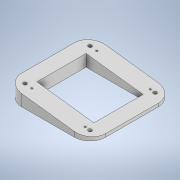
# Autodesk Inventor part: 頸部桌面轉接件
Saved by Autodesk Inventor 2021 (Build 250183000, 183)
## iProperties
Created: 2023-02-10
Part Number: 頸部桌面轉接件
Material: 一般
Document SubType Name: Modeling
Designer: brian
Density: 1 g/cm^3
Appearance: 預設
Author: brian
Autodesk Inventor part; units mm, degrees
ref_plane "YZ Plane" through (0, 0, 0) normal (1, 0, 0) x (0, 1, 0)
ref_plane "XZ Plane" through (0, 0, 0) normal (0, 1, 0) x (-1, 0, 0)
sketch "草圖1" plane through (0, 0, 0) normal (0, 1, 0) x (-1, 0, 0)
  line L0 (132.5, 132.5) -> (-132.5, 132.5)
  line L1 (-132.5, 132.5) -> (-132.5, -132.5)
  line L2 (-132.5, -132.5) -> (132.5, -132.5)
  line L3 (132.5, -132.5) -> (132.5, 132.5)
  line L4 (132.5, 132.5) -> (-132.5, -132.5) construction
  line L5 (-132.5, 132.5) -> (132.5, -132.5) construction
  point P0 (0, 0)
  dimension "d0" = 265
  dimension "d1" = 265
  constraints: 12 end point, 2 midpoint, 2 parallel, 1 horizontal, 1 perpendicular
  measures "d0" distance of L1.end L2.end
  measures "d1" distance of L0.end L1.end
extrude "擠出1" add sketch "草圖1" along normal blind 10
sketch "草圖3" plane through (0, 10, 0) normal (0, 1, 0) x (1, 0, 0)
  line L0 (132.5, -132.5) -> (132.5, 132.5) projected
  line L1 (132.5, 132.5) -> (-132.5, 132.5) projected
  line L2 (-132.5, 132.5) -> (-132.5, -132.5) projected
  line L3 (-132.5, -132.5) -> (132.5, -132.5) projected
  point P0 (0, 0)
extrude "擠出2" add sketch "草圖3" along normal blind 100
sketch "草圖4" plane through (132.5, 0, 132.5) normal (1, 0, 0) x (0, 0, -1)
  line L0 (0, 0) -> (265, 0) projected
  line L1 (265, 0) -> (265, 110) projected
  line L2 (0, 110) -> (265, 110) projected
  line L3 (0, 0) -> (0, 110) projected
  line L4 (0, 0) -> (0, 110) projected
  line L5 (0, 10) -> (265, 10)
  point P0 (132.5, 0)
  dimension "d7" = 10
  constraints: 2 end point, 2 point on line, 1 perpendicular
  measures "d7" distance between parallel lines of L0 L5
ref_plane "工作平面2" through (132.5, 10, 132.5) normal (0.1218693, 0.9925462, 0) x (0, 0, -1)
split "分割1" plane through (132.5, 10, 132.5) removes the side toward (0.1218693, 0.9925462, 0)
sketch "草圖5" plane through (0, 0, 0) normal (0, -1, 0) x (1, 0, 0)
  line L0 (-102.5, -102.5) -> (102.5, -102.5) construction
  line L1 (102.5, -102.5) -> (102.5, 102.5) construction
  line L2 (102.5, 102.5) -> (-102.5, 102.5) construction
  line L3 (-102.5, 102.5) -> (-102.5, -102.5) construction
  line L4 (-102.5, -102.5) -> (102.5, 102.5) construction
  line L5 (102.5, -102.5) -> (-102.5, 102.5) construction
  point P0 (0, 0)
  dimension "d9" = 205
  dimension "d10" = 205
  constraints: 12 end point, 4 coincident, 2 midpoint, 2 parallel, 1 horizontal, 1 perpendicular
  measures "d9" distance of L2.end L1.end
  measures "d10" distance of L1.end L0.end
hole "孔1" at (-102.5, 0, -102.5) at (102.5, 0, -102.5) at (102.5, 0, 102.5) at (-102.5, 0, 102.5) direction (0, 1, 0) diameter 5.5 depth 8
sketch "草圖6" plane through (-102.5, 8, -102.5) normal (0, -1, 0) x (1, 0, 0)
  circle A0 centre (0, 205) radius 2.75 projected
  circle A1 centre (205, 205) radius 2.75 projected
  circle A2 centre (205, 0) radius 2.75 projected
  circle A3 centre (0, 0) radius 2.75 projected
  circle A4 centre (0, 0) radius 2.75 projected
  circle A5 centre (205, 0) radius 2.75 projected
  circle A6 centre (0, 205) radius 2.75 projected
  point P0 (102.5, 102.5)
  constraints: 4 coincident
hole "孔2" at (-102.5, 8, -102.5) at (102.5, 8, -102.5) at (102.5, 8, 102.5) at (-102.5, 8, 102.5) direction (0, 1, 0) diameter 11 end through all
sketch "草圖7" plane through (132.5, 10, 132.5) normal (0.1218693, 0.9925462, 0) x (0.9925462, -0.1218693, 0)
  line L0 (-215.2937, 30) -> (-45.2937, 30)
  line L1 (-45.2937, 30) -> (-45.2937, 235)
  line L2 (-45.2937, 235) -> (-215.2937, 235)
  line L3 (-215.2937, 235) -> (-215.2937, 30)
  line L4 (-215.2937, 30) -> (-45.2937, 235) construction
  line L5 (-45.2937, 30) -> (-215.2937, 235) construction
  point P0 (-130.2937, 132.5)
  dimension "d25" = 170
  dimension "d26" = 205
  constraints: 12 end point, 4 coincident, 2 midpoint, 2 parallel, 1 horizontal, 1 perpendicular
  measures "d25" distance of L2.end L1.end
  measures "d26" distance of L1.end L0.end
hole "孔3" at (-81.1889, 36.2377, 102.5) at (87.5439, 15.5199, 102.5) at (87.5439, 15.5199, -102.5) at (-81.1889, 36.2377, -102.5) direction (-0.1218693, -0.9925462, 0) diameter 3.5 depth 13 counterbore diameter 5.8 counterbore depth 8.6
sketch "草圖8" plane through (0, 0, 0) normal (0, -1, 0) x (1, 0, 0)
  line L0 (-90, 77.5) -> (90, 77.5)
  line L1 (90, 77.5) -> (90, -77.5)
  line L2 (90, -77.5) -> (-90, -77.5)
  line L3 (-90, -77.5) -> (-90, 77.5)
  line L4 (-90, 77.5) -> (90, -77.5) construction
  line L5 (90, 77.5) -> (-90, -77.5) construction
  point P0 (0, 0)
  dimension "d34" = 180
  dimension "d35" = 155
  constraints: 12 end point, 2 midpoint, 2 parallel, 1 horizontal, 1 perpendicular
  measures "d34" distance of L1.end L2.end
  measures "d35" distance of L0.end L1.end
extrude "擠出3" cut sketch "草圖8" against normal through all
fillet "圓角1" radius 50 4 edges at (-132.5, 21.269, 132.5) (-132.5, 21.269, -132.5) (132.5, 5, -132.5) (132.5, 5, 132.5)
